Autodesk Inventor part; units mm, degrees
(part 8 of 13)
  line L2760 (6.8105, 15.183) -> (1.0789, 15.183)
  arc A2760 (1.0789, 15.183) -> (1.0789, 15.057) centre (1.0789, 15.12) ccw
  line L2761 (8.5894, 15.057) -> (17.121, 15.057)
  arc A2761 (17.121, 15.057) -> (17.121, 15.183) centre (17.121, 15.12) ccw
  line L2762 (17.121, 15.183) -> (8.5894, 15.183)
  arc A2762 (8.5894, 15.183) -> (8.5894, 15.057) centre (8.5894, 15.12) ccw
  line L2763 (1.0789, 15.183) -> (6.9365, 15.183)
  arc A2763 (6.9365, 15.183) -> (6.9365, 15.309) centre (6.9365, 15.246) ccw
  line L2764 (6.9365, 15.309) -> (1.0789, 15.309)
  arc A2764 (1.0789, 15.309) -> (1.0789, 15.183) centre (1.0789, 15.246) ccw
  line L2765 (8.4634, 15.183) -> (17.121, 15.183)
  arc A2765 (17.121, 15.183) -> (17.121, 15.309) centre (17.121, 15.246) ccw
  line L2766 (17.121, 15.309) -> (8.4634, 15.309)
  arc A2766 (8.4634, 15.309) -> (8.4634, 15.183) centre (8.4634, 15.246) ccw
  line L2767 (1.0789, 15.309) -> (7.1747, 15.309)
  arc A2767 (7.1747, 15.309) -> (7.1747, 15.435) centre (7.1747, 15.372) ccw
  line L2768 (7.1747, 15.435) -> (1.0789, 15.435)
  arc A2768 (1.0789, 15.435) -> (1.0789, 15.309) centre (1.0789, 15.372) ccw
  line L2769 (8.2253, 15.309) -> (17.121, 15.309)
  arc A2769 (17.121, 15.309) -> (17.121, 15.435) centre (17.121, 15.372) ccw
  line L2770 (17.121, 15.435) -> (8.2253, 15.435)
  arc A2770 (8.2253, 15.435) -> (8.2253, 15.309) centre (8.2253, 15.372) ccw
  line L2771 (1.0789, 15.435) -> (17.121, 15.435)
  arc A2771 (17.121, 15.435) -> (17.121, 15.561) centre (17.121, 15.498) ccw
  line L2772 (17.121, 15.561) -> (1.0789, 15.561)
  arc A2772 (1.0789, 15.561) -> (1.0789, 15.435) centre (1.0789, 15.498) ccw
  line L2773 (1.0789, 15.561) -> (17.121, 15.561)
  arc A2773 (17.121, 15.561) -> (17.121, 15.687) centre (17.121, 15.624) ccw
  line L2774 (17.121, 15.687) -> (1.0789, 15.687)
  arc A2774 (1.0789, 15.687) -> (1.0789, 15.561) centre (1.0789, 15.624) ccw
  line L2775 (1.0789, 15.687) -> (17.121, 15.687)
  arc A2775 (17.121, 15.687) -> (17.121, 15.813) centre (17.121, 15.75) ccw
  line L2776 (17.121, 15.813) -> (1.0789, 15.813)
  arc A2776 (1.0789, 15.813) -> (1.0789, 15.687) centre (1.0789, 15.75) ccw
  line L2777 (1.0789, 15.813) -> (17.121, 15.813)
  arc A2777 (17.121, 15.813) -> (17.121, 15.939) centre (17.121, 15.876) ccw
  line L2778 (17.121, 15.939) -> (1.0789, 15.939)
  arc A2778 (1.0789, 15.939) -> (1.0789, 15.813) centre (1.0789, 15.876) ccw
  line L2779 (1.0789, 15.939) -> (17.121, 15.939)
  arc A2779 (17.121, 15.939) -> (17.121, 16.065) centre (17.121, 16.002) ccw
  line L2780 (17.121, 16.065) -> (1.0789, 16.065)
  arc A2780 (1.0789, 16.065) -> (1.0789, 15.939) centre (1.0789, 16.002) ccw
  line L2781 (1.0789, 16.065) -> (17.121, 16.065)
  arc A2781 (17.121, 16.065) -> (17.121, 16.191) centre (17.121, 16.128) ccw
  line L2782 (17.121, 16.191) -> (1.0789, 16.191)
  arc A2782 (1.0789, 16.191) -> (1.0789, 16.065) centre (1.0789, 16.128) ccw
  line L2783 (1.0789, 16.191) -> (17.121, 16.191)
  arc A2783 (17.121, 16.191) -> (17.121, 16.317) centre (17.121, 16.254) ccw
  line L2784 (17.121, 16.317) -> (1.0789, 16.317)
  arc A2784 (1.0789, 16.317) -> (1.0789, 16.191) centre (1.0789, 16.254) ccw
  line L2785 (1.0789, 16.317) -> (17.121, 16.317)
  arc A2785 (17.121, 16.317) -> (17.121, 16.443) centre (17.121, 16.38) ccw
  line L2786 (17.121, 16.443) -> (1.0789, 16.443)
  arc A2786 (1.0789, 16.443) -> (1.0789, 16.317) centre (1.0789, 16.38) ccw
  line L2787 (1.0789, 16.443) -> (17.121, 16.443)
  arc A2787 (17.121, 16.443) -> (17.121, 16.569) centre (17.121, 16.506) ccw
  line L2788 (17.121, 16.569) -> (1.0789, 16.569)
  arc A2788 (1.0789, 16.569) -> (1.0789, 16.443) centre (1.0789, 16.506) ccw
  line L2789 (1.0789, 16.569) -> (17.121, 16.569)
  arc A2789 (17.121, 16.569) -> (17.121, 16.695) centre (17.121, 16.632) ccw
  line L2790 (17.121, 16.695) -> (1.0789, 16.695)
  arc A2790 (1.0789, 16.695) -> (1.0789, 16.569) centre (1.0789, 16.632) ccw
  line L2791 (1.0789, 16.695) -> (17.121, 16.695)
  arc A2791 (17.121, 16.695) -> (17.121, 16.821) centre (17.121, 16.758) ccw
  line L2792 (17.121, 16.821) -> (1.0789, 16.821)
  arc A2792 (1.0789, 16.821) -> (1.0789, 16.695) centre (1.0789, 16.758) ccw
  line L2793 (1.0789, 16.821) -> (17.121, 16.821)
  arc A2793 (17.121, 16.821) -> (17.121, 16.947) centre (17.121, 16.884) ccw
  line L2794 (17.121, 16.947) -> (1.0789, 16.947)
  arc A2794 (1.0789, 16.947) -> (1.0789, 16.821) centre (1.0789, 16.884) ccw
  line L2795 (1.0789, 16.947) -> (17.121, 16.947)
  arc A2795 (17.121, 16.947) -> (17.121, 17.073) centre (17.121, 17.01) ccw
  line L2796 (17.121, 17.073) -> (1.0789, 17.073)
  arc A2796 (1.0789, 17.073) -> (1.0789, 16.947) centre (1.0789, 17.01) ccw
  line L2797 (1.0789, 17.073) -> (17.121, 17.073)
  arc A2797 (17.121, 17.073) -> (17.121, 17.199) centre (17.121, 17.136) ccw
  line L2798 (17.121, 17.199) -> (1.0789, 17.199)
  arc A2798 (1.0789, 17.199) -> (1.0789, 17.073) centre (1.0789, 17.136) ccw
  line L2799 (1.0789, 17.199) -> (17.121, 17.199)
  arc A2799 (17.121, 17.199) -> (17.121, 17.325) centre (17.121, 17.262) ccw
  line L2800 (17.121, 17.325) -> (1.0789, 17.325)
  arc A2800 (1.0789, 17.325) -> (1.0789, 17.199) centre (1.0789, 17.262) ccw
  line L2801 (1.0789, 17.325) -> (17.121, 17.325)
  arc A2801 (17.121, 17.325) -> (17.121, 17.451) centre (17.121, 17.388) ccw
  line L2802 (17.121, 17.451) -> (1.0789, 17.451)
  arc A2802 (1.0789, 17.451) -> (1.0789, 17.325) centre (1.0789, 17.388) ccw
  line L2803 (1.0789, 17.451) -> (17.121, 17.451)
  arc A2803 (17.121, 17.451) -> (17.121, 17.577) centre (17.121, 17.514) ccw
  line L2804 (17.121, 17.577) -> (1.0789, 17.577)
  arc A2804 (1.0789, 17.577) -> (1.0789, 17.451) centre (1.0789, 17.514) ccw
  line L2805 (1.0789, 17.577) -> (17.121, 17.577)
  arc A2805 (17.121, 17.577) -> (17.121, 17.703) centre (17.121, 17.64) ccw
  line L2806 (17.121, 17.703) -> (1.0789, 17.703)
  arc A2806 (1.0789, 17.703) -> (1.0789, 17.577) centre (1.0789, 17.64) ccw
  line L2807 (1.0789, 17.703) -> (17.121, 17.703)
  arc A2807 (17.121, 17.703) -> (17.121, 17.829) centre (17.121, 17.766) ccw
  line L2808 (17.121, 17.829) -> (1.0789, 17.829)
  arc A2808 (1.0789, 17.829) -> (1.0789, 17.703) centre (1.0789, 17.766) ccw
  line L2809 (1.0789, 17.829) -> (17.121, 17.829)
  arc A2809 (17.121, 17.829) -> (17.121, 17.955) centre (17.121, 17.892) ccw
  line L2810 (17.121, 17.955) -> (1.0789, 17.955)
  arc A2810 (1.0789, 17.955) -> (1.0789, 17.829) centre (1.0789, 17.892) ccw
  line L2811 (1.0789, 17.955) -> (7.2227, 17.955)
  arc A2811 (7.2227, 17.955) -> (7.2227, 18.081) centre (7.2227, 18.018) ccw
  line L2812 (7.2227, 18.081) -> (1.0789, 18.081)
  arc A2812 (1.0789, 18.081) -> (1.0789, 17.955) centre (1.0789, 18.018) ccw
  line L2813 (7.637, 17.955) -> (7.7628, 17.955)
  arc A2813 (7.7628, 17.955) -> (7.7628, 18.081) centre (7.7628, 18.018) ccw
  line L2814 (7.7628, 18.081) -> (7.637, 18.081)
  arc A2814 (7.637, 18.081) -> (7.637, 17.955) centre (7.637, 18.018) ccw
  line L2815 (8.1771, 17.955) -> (17.121, 17.955)
  arc A2815 (17.121, 17.955) -> (17.121, 18.081) centre (17.121, 18.018) ccw
  line L2816 (17.121, 18.081) -> (8.1771, 18.081)
  arc A2816 (8.1771, 18.081) -> (8.1771, 17.955) centre (8.1771, 18.018) ccw
  line L2817 (1.0789, 18.081) -> (6.9227, 18.081)
  arc A2817 (6.9227, 18.081) -> (6.9227, 18.207) centre (6.9227, 18.144) ccw
  line L2818 (6.9227, 18.207) -> (1.0789, 18.207)
  arc A2818 (1.0789, 18.207) -> (1.0789, 18.081) centre (1.0789, 18.144) ccw
  line L2819 (7.637, 18.081) -> (7.7628, 18.081)
  arc A2819 (7.7628, 18.081) -> (7.7628, 18.207) centre (7.7628, 18.144) ccw
  line L2820 (7.7628, 18.207) -> (7.637, 18.207)
  arc A2820 (7.637, 18.207) -> (7.637, 18.081) centre (7.637, 18.144) ccw
  line L2821 (8.4772, 18.081) -> (17.121, 18.081)
  arc A2821 (17.121, 18.081) -> (17.121, 18.207) centre (17.121, 18.144) ccw
  line L2822 (17.121, 18.207) -> (8.4772, 18.207)
  arc A2822 (8.4772, 18.207) -> (8.4772, 18.081) centre (8.4772, 18.144) ccw
  line L2823 (1.0789, 18.207) -> (6.7967, 18.207)
  arc A2823 (6.7967, 18.207) -> (6.7967, 18.333) centre (6.7967, 18.27) ccw
  line L2824 (6.7967, 18.333) -> (1.0789, 18.333)
  arc A2824 (1.0789, 18.333) -> (1.0789, 18.207) centre (1.0789, 18.27) ccw
  line L2825 (7.637, 18.207) -> (7.7628, 18.207)
  arc A2825 (7.7628, 18.207) -> (7.7628, 18.333) centre (7.7628, 18.27) ccw
  line L2826 (7.7628, 18.333) -> (7.637, 18.333)
  arc A2826 (7.637, 18.333) -> (7.637, 18.207) centre (7.637, 18.27) ccw
  line L2827 (8.6032, 18.207) -> (17.121, 18.207)
  arc A2827 (17.121, 18.207) -> (17.121, 18.333) centre (17.121, 18.27) ccw
  line L2828 (17.121, 18.333) -> (8.6032, 18.333)
  arc A2828 (8.6032, 18.333) -> (8.6032, 18.207) centre (8.6032, 18.27) ccw
  line L2829 (1.0789, 18.333) -> (1.3493, 18.333)
  arc A2829 (1.3493, 18.333) -> (1.3493, 18.459) centre (1.3493, 18.396) ccw
  line L2830 (1.3493, 18.459) -> (1.0789, 18.459)
  arc A2830 (1.0789, 18.459) -> (1.0789, 18.333) centre (1.0789, 18.396) ccw
  line L2831 (3.4506, 18.333) -> (6.6707, 18.333)
  arc A2831 (6.6707, 18.333) -> (6.6707, 18.459) centre (6.6707, 18.396) ccw
  line L2832 (6.6707, 18.459) -> (3.4506, 18.459)
  arc A2832 (3.4506, 18.459) -> (3.4506, 18.333) centre (3.4506, 18.396) ccw
  line L2833 (7.637, 18.333) -> (7.7628, 18.333)
  arc A2833 (7.7628, 18.333) -> (7.7628, 18.459) centre (7.7628, 18.396) ccw
  line L2834 (7.7628, 18.459) -> (7.637, 18.459)
  arc A2834 (7.637, 18.459) -> (7.637, 18.333) centre (7.637, 18.396) ccw
  line L2835 (8.7292, 18.333) -> (17.121, 18.333)
  arc A2835 (17.121, 18.333) -> (17.121, 18.459) centre (17.121, 18.396) ccw
  line L2836 (17.121, 18.459) -> (8.7292, 18.459)
  arc A2836 (8.7292, 18.459) -> (8.7292, 18.333) centre (8.7292, 18.396) ccw
  line L2837 (1.0789, 18.459) -> (1.2846, 18.459)
  arc A2837 (1.2846, 18.459) -> (1.2846, 18.585) centre (1.2846, 18.522) ccw
  line L2838 (1.2846, 18.585) -> (1.0789, 18.585)
  arc A2838 (1.0789, 18.585) -> (1.0789, 18.459) centre (1.0789, 18.522) ccw
  line L2839 (3.5153, 18.459) -> (6.5447, 18.459)
  arc A2839 (6.5447, 18.459) -> (6.5447, 18.585) centre (6.5447, 18.522) ccw
  line L2840 (6.5447, 18.585) -> (3.5153, 18.585)
  arc A2840 (3.5153, 18.585) -> (3.5153, 18.459) centre (3.5153, 18.522) ccw
  line L2841 (7.637, 18.459) -> (7.7628, 18.459)
  arc A2841 (7.7628, 18.459) -> (7.7628, 18.585) centre (7.7628, 18.522) ccw
  line L2842 (7.7628, 18.585) -> (7.637, 18.585)
  arc A2842 (7.637, 18.585) -> (7.637, 18.459) centre (7.637, 18.522) ccw
  line L2843 (8.8552, 18.459) -> (17.121, 18.459)
  arc A2843 (17.121, 18.459) -> (17.121, 18.585) centre (17.121, 18.522) ccw
  line L2844 (17.121, 18.585) -> (8.8552, 18.585)
  arc A2844 (8.8552, 18.585) -> (8.8552, 18.459) centre (8.8552, 18.522) ccw
  line L2845 (1.0789, 18.585) -> (1.2846, 18.585)
  arc A2845 (1.2846, 18.585) -> (1.2846, 18.711) centre (1.2846, 18.648) ccw
  line L2846 (1.2846, 18.711) -> (1.0789, 18.711)
  arc A2846 (1.0789, 18.711) -> (1.0789, 18.585) centre (1.0789, 18.648) ccw
  line L2847 (3.5153, 18.585) -> (6.4904, 18.585)
  arc A2847 (6.4904, 18.585) -> (6.4904, 18.711) centre (6.4904, 18.648) ccw
  line L2848 (6.4904, 18.711) -> (3.5153, 18.711)
  arc A2848 (3.5153, 18.711) -> (3.5153, 18.585) centre (3.5153, 18.648) ccw
  line L2849 (7.637, 18.585) -> (7.7628, 18.585)
  arc A2849 (7.7628, 18.585) -> (7.7628, 18.711) centre (7.7628, 18.648) ccw
  line L2850 (7.7628, 18.711) -> (7.637, 18.711)
  arc A2850 (7.637, 18.711) -> (7.637, 18.585) centre (7.637, 18.648) ccw
  line L2851 (8.9094, 18.585) -> (17.121, 18.585)
  arc A2851 (17.121, 18.585) -> (17.121, 18.711) centre (17.121, 18.648) ccw
  line L2852 (17.121, 18.711) -> (8.9094, 18.711)
  arc A2852 (8.9094, 18.711) -> (8.9094, 18.585) centre (8.9094, 18.648) ccw
  line L2853 (1.0789, 18.711) -> (1.2846, 18.711)
  arc A2853 (1.2846, 18.711) -> (1.2846, 18.837) centre (1.2846, 18.774) ccw
  line L2854 (1.2846, 18.837) -> (1.0789, 18.837)
  arc A2854 (1.0789, 18.837) -> (1.0789, 18.711) centre (1.0789, 18.774) ccw
  line L2855 (3.5153, 18.711) -> (6.4382, 18.711)
  arc A2855 (6.4382, 18.711) -> (6.4382, 18.837) centre (6.4382, 18.774) ccw
  line L2856 (6.4382, 18.837) -> (3.5153, 18.837)
  arc A2856 (3.5153, 18.837) -> (3.5153, 18.711) centre (3.5153, 18.774) ccw
  line L2857 (7.637, 18.711) -> (7.7628, 18.711)
  arc A2857 (7.7628, 18.711) -> (7.7628, 18.837) centre (7.7628, 18.774) ccw
  line L2858 (7.7628, 18.837) -> (7.637, 18.837)
  arc A2858 (7.637, 18.837) -> (7.637, 18.711) centre (7.637, 18.774) ccw
  line L2859 (8.9616, 18.711) -> (17.121, 18.711)
  arc A2859 (17.121, 18.711) -> (17.121, 18.837) centre (17.121, 18.774) ccw
  line L2860 (17.121, 18.837) -> (8.9616, 18.837)
  arc A2860 (8.9616, 18.837) -> (8.9616, 18.711) centre (8.9616, 18.774) ccw
  line L2861 (1.0789, 18.837) -> (1.2846, 18.837)
  arc A2861 (1.2846, 18.837) -> (1.2846, 18.963) centre (1.2846, 18.9) ccw
  line L2862 (1.2846, 18.963) -> (1.0789, 18.963)
  arc A2862 (1.0789, 18.963) -> (1.0789, 18.837) centre (1.0789, 18.9) ccw
  line L2863 (3.5153, 18.837) -> (6.386, 18.837)
  arc A2863 (6.386, 18.837) -> (6.386, 18.963) centre (6.386, 18.9) ccw
  line L2864 (6.386, 18.963) -> (3.5153, 18.963)
  arc A2864 (3.5153, 18.963) -> (3.5153, 18.837) centre (3.5153, 18.9) ccw
  line L2865 (7.637, 18.837) -> (7.7628, 18.837)
  arc A2865 (7.7628, 18.837) -> (7.7628, 18.963) centre (7.7628, 18.9) ccw
  line L2866 (7.7628, 18.963) -> (7.637, 18.963)
  arc A2866 (7.637, 18.963) -> (7.637, 18.837) centre (7.637, 18.9) ccw
  line L2867 (9.0138, 18.837) -> (17.121, 18.837)
  arc A2867 (17.121, 18.837) -> (17.121, 18.963) centre (17.121, 18.9) ccw
  line L2868 (17.121, 18.963) -> (9.0138, 18.963)
  arc A2868 (9.0138, 18.963) -> (9.0138, 18.837) centre (9.0138, 18.9) ccw
  line L2869 (1.0789, 18.963) -> (1.2846, 18.963)
  arc A2869 (1.2846, 18.963) -> (1.2846, 19.089) centre (1.2846, 19.026) ccw
  line L2870 (1.2846, 19.089) -> (1.0789, 19.089)
  arc A2870 (1.0789, 19.089) -> (1.0789, 18.963) centre (1.0789, 19.026) ccw
  line L2871 (3.5153, 18.963) -> (6.3338, 18.963)
  arc A2871 (6.3338, 18.963) -> (6.3338, 19.089) centre (6.3338, 19.026) ccw
  line L2872 (6.3338, 19.089) -> (3.5153, 19.089)
  arc A2872 (3.5153, 19.089) -> (3.5153, 18.963) centre (3.5153, 19.026) ccw
  line L2873 (7.637, 18.963) -> (7.7628, 18.963)
  arc A2873 (7.7628, 18.963) -> (7.7632, 19.089) centre (7.763, 19.026) ccw
  line L2874 (7.7632, 19.089) -> (7.6374, 19.089)
  arc A2874 (7.6374, 19.089) -> (7.637, 18.963) centre (7.6372, 19.026) ccw
  line L2875 (9.066, 18.963) -> (17.121, 18.963)
  arc A2875 (17.121, 18.963) -> (17.1212, 19.0315) centre (17.174, 18.9971) ccw
  line L2876 (17.1212, 19.0315) -> (9.0664, 19.089)
  arc A2876 (9.0664, 19.089) -> (9.066, 18.963) centre (9.0662, 19.026) ccw
  line L2877 (1.0789, 19.089) -> (1.2846, 19.089)
  arc A2877 (1.2846, 19.089) -> (1.2846, 19.215) centre (1.2846, 19.152) ccw
  line L2878 (1.2846, 19.215) -> (1.0789, 19.215)
  arc A2878 (1.0789, 19.215) -> (1.0789, 19.089) centre (1.0789, 19.152) ccw
  line L2879 (3.5153, 19.089) -> (6.333, 19.089)
  arc A2879 (6.333, 19.089) -> (6.3334, 19.215) centre (6.3334, 19.152) ccw
  line L2880 (6.3334, 19.215) -> (3.5157, 19.215)
  arc A2880 (3.5157, 19.215) -> (3.5153, 19.089) centre (3.5155, 19.152) ccw
  line L2881 (7.6374, 19.089) -> (7.7632, 19.089)
  arc A2881 (7.7632, 19.089) -> (7.7632, 19.215) centre (7.7632, 19.152) ccw
  line L2882 (7.7632, 19.215) -> (7.6374, 19.215)
  arc A2882 (7.6374, 19.215) -> (7.6374, 19.089) centre (7.6374, 19.152) ccw
  line L2883 (9.0673, 19.089) -> (17.1212, 19.0315)
  arc A2883 (17.1212, 19.0315) -> (17.1214, 19.215) centre (17.1213, 19.1232) ccw
  line L2884 (17.1214, 19.215) -> (9.0673, 19.215)
  arc A2884 (9.0673, 19.215) -> (9.0673, 19.089) centre (9.0673, 19.152) ccw
  line L2885 (1.0789, 19.215) -> (1.2846, 19.215)
  arc A2885 (1.2846, 19.215) -> (1.2846, 19.341) centre (1.2846, 19.278) ccw
  line L2886 (1.2846, 19.341) -> (1.0789, 19.341)
  arc A2886 (1.0789, 19.341) -> (1.0789, 19.215) centre (1.0789, 19.278) ccw
  line L2887 (3.5157, 19.215) -> (7.6369, 19.215)
  arc A2887 (7.6369, 19.215) -> (7.6369, 19.341) centre (7.6369, 19.278) ccw
  line L2888 (7.6369, 19.341) -> (3.5157, 19.341)
  arc A2888 (3.5157, 19.341) -> (3.5157, 19.215) centre (3.5157, 19.278) ccw
  line L2889 (7.7638, 19.215) -> (17.1214, 19.215)
  arc A2889 (17.1214, 19.215) -> (17.1214, 19.341) centre (17.1214, 19.278) ccw
  line L2890 (17.1214, 19.341) -> (7.7638, 19.341)
  arc A2890 (7.7638, 19.341) -> (7.7638, 19.215) centre (7.7638, 19.278) ccw
  line L2891 (1.0789, 19.341) -> (1.2846, 19.341)
  arc A2891 (1.2846, 19.341) -> (1.2846, 19.467) centre (1.2846, 19.404) ccw
  line L2892 (1.2846, 19.467) -> (1.0789, 19.467)
  arc A2892 (1.0789, 19.467) -> (1.0789, 19.341) centre (1.0789, 19.404) ccw
  line L2893 (3.5157, 19.341) -> (6.3334, 19.341)
  arc A2893 (6.3334, 19.341) -> (6.3334, 19.467) centre (6.3334, 19.404) ccw
  line L2894 (6.3334, 19.467) -> (3.5157, 19.467)
  arc A2894 (3.5157, 19.467) -> (3.5157, 19.341) centre (3.5157, 19.404) ccw
  line L2895 (7.6374, 19.341) -> (7.7632, 19.341)
  arc A2895 (7.7632, 19.341) -> (7.7632, 19.467) centre (7.7632, 19.404) ccw
  line L2896 (7.7632, 19.467) -> (7.6374, 19.467)
  arc A2896 (7.6374, 19.467) -> (7.6374, 19.341) centre (7.6374, 19.404) ccw
  line L2897 (9.0673, 19.341) -> (17.1214, 19.341)
  arc A2897 (17.1214, 19.341) -> (17.1214, 19.467) centre (17.1214, 19.404) ccw
  line L2898 (17.1214, 19.467) -> (9.0673, 19.467)
  arc A2898 (9.0673, 19.467) -> (9.0673, 19.341) centre (9.0673, 19.404) ccw
  line L2899 (1.0789, 19.467) -> (1.2846, 19.467)
  arc A2899 (1.2846, 19.467) -> (1.2846, 19.593) centre (1.2846, 19.53) ccw
  line L2900 (1.2846, 19.593) -> (1.0789, 19.593)
  arc A2900 (1.0789, 19.593) -> (1.0789, 19.467) centre (1.0789, 19.53) ccw
  line L2901 (3.5157, 19.467) -> (6.3334, 19.467)
  arc A2901 (6.3334, 19.467) -> (6.3334, 19.593) centre (6.3334, 19.53) ccw
  line L2902 (6.3334, 19.593) -> (3.5157, 19.593)
  arc A2902 (3.5157, 19.593) -> (3.5157, 19.467) centre (3.5157, 19.53) ccw
  line L2903 (7.6374, 19.467) -> (7.7632, 19.467)
  arc A2903 (7.7632, 19.467) -> (7.7632, 19.593) centre (7.7632, 19.53) ccw
  line L2904 (7.7632, 19.593) -> (7.6374, 19.593)
  arc A2904 (7.6374, 19.593) -> (7.6374, 19.467) centre (7.6374, 19.53) ccw
  line L2905 (9.0673, 19.467) -> (17.1214, 19.467)
  arc A2905 (17.1214, 19.467) -> (17.121, 19.593) centre (17.1212, 19.53) ccw
  line L2906 (17.121, 19.593) -> (9.0669, 19.593)
  arc A2906 (9.0669, 19.593) -> (9.0673, 19.467) centre (9.0671, 19.53) ccw
  line L2907 (1.0789, 19.593) -> (1.2846, 19.593)
  arc A2907 (1.2846, 19.593) -> (1.2846, 19.719) centre (1.2846, 19.656) ccw
  line L2908 (1.2846, 19.719) -> (1.0789, 19.719)
  arc A2908 (1.0789, 19.719) -> (1.0789, 19.593) centre (1.0789, 19.656) ccw
  line L2909 (3.5157, 19.593) -> (6.3683, 19.593)
  arc A2909 (6.3683, 19.593) -> (6.3683, 19.719) centre (6.3683, 19.656) ccw
  line L2910 (6.3683, 19.719) -> (3.5157, 19.719)
  arc A2910 (3.5157, 19.719) -> (3.5157, 19.593) centre (3.5157, 19.656) ccw
  line L2911 (7.6374, 19.593) -> (7.7632, 19.593)
  arc A2911 (7.7632, 19.593) -> (7.7632, 19.719) centre (7.7632, 19.656) ccw
  line L2912 (7.7632, 19.719) -> (7.6374, 19.719)
  arc A2912 (7.6374, 19.719) -> (7.6374, 19.593) centre (7.6374, 19.656) ccw
  line L2913 (9.0321, 19.593) -> (17.121, 19.593)
  arc A2913 (17.121, 19.593) -> (17.121, 19.719) centre (17.121, 19.656) ccw
  line L2914 (17.121, 19.719) -> (9.0321, 19.719)
  arc A2914 (9.0321, 19.719) -> (9.0321, 19.593) centre (9.0321, 19.656) ccw
  line L2915 (1.0789, 19.719) -> (1.2846, 19.719)
  arc A2915 (1.2846, 19.719) -> (1.2846, 19.845) centre (1.2846, 19.782) ccw
  line L2916 (1.2846, 19.845) -> (1.0789, 19.845)
  arc A2916 (1.0789, 19.845) -> (1.0789, 19.719) centre (1.0789, 19.782) ccw
  line L2917 (3.5157, 19.719) -> (6.4205, 19.719)
  arc A2917 (6.4205, 19.719) -> (6.4205, 19.845) centre (6.4205, 19.782) ccw
  line L2918 (6.4205, 19.845) -> (3.5157, 19.845)
  arc A2918 (3.5157, 19.845) -> (3.5157, 19.719) centre (3.5157, 19.782) ccw
  line L2919 (7.6374, 19.719) -> (7.7632, 19.719)
  arc A2919 (7.7632, 19.719) -> (7.7632, 19.845) centre (7.7632, 19.782) ccw
  line L2920 (7.7632, 19.845) -> (7.6374, 19.845)
  arc A2920 (7.6374, 19.845) -> (7.6374, 19.719) centre (7.6374, 19.782) ccw
  line L2921 (8.9799, 19.719) -> (17.121, 19.719)
  arc A2921 (17.121, 19.719) -> (17.121, 19.845) centre (17.121, 19.782) ccw
  line L2922 (17.121, 19.845) -> (8.9799, 19.845)
  arc A2922 (8.9799, 19.845) -> (8.9799, 19.719) centre (8.9799, 19.782) ccw
  line L2923 (1.0789, 19.845) -> (1.2846, 19.845)
  arc A2923 (1.2846, 19.845) -> (1.2846, 19.971) centre (1.2846, 19.908) ccw
  line L2924 (1.2846, 19.971) -> (1.0789, 19.971)
  arc A2924 (1.0789, 19.971) -> (1.0789, 19.845) centre (1.0789, 19.908) ccw
  line L2925 (3.5157, 19.845) -> (6.4727, 19.845)
  arc A2925 (6.4727, 19.845) -> (6.4727, 19.971) centre (6.4727, 19.908) ccw
  line L2926 (6.4727, 19.971) -> (3.5157, 19.971)
  arc A2926 (3.5157, 19.971) -> (3.5157, 19.845) centre (3.5157, 19.908) ccw
  line L2927 (7.6374, 19.845) -> (7.7632, 19.845)
  arc A2927 (7.7632, 19.845) -> (7.7632, 19.971) centre (7.7632, 19.908) ccw
  line L2928 (7.7632, 19.971) -> (7.6374, 19.971)
  arc A2928 (7.6374, 19.971) -> (7.6374, 19.845) centre (7.6374, 19.908) ccw
  line L2929 (8.9277, 19.845) -> (17.121, 19.845)
  arc A2929 (17.121, 19.845) -> (17.121, 19.971) centre (17.121, 19.908) ccw
  line L2930 (17.121, 19.971) -> (8.9277, 19.971)
  arc A2930 (8.9277, 19.971) -> (8.9277, 19.845) centre (8.9277, 19.908) ccw
  line L2931 (1.0789, 19.971) -> (1.2846, 19.971)
  arc A2931 (1.2846, 19.971) -> (1.2846, 20.097) centre (1.2846, 20.034) ccw
  line L2932 (1.2846, 20.097) -> (1.0789, 20.097)
  arc A2932 (1.0789, 20.097) -> (1.0789, 19.971) centre (1.0789, 20.034) ccw
  line L2933 (3.5157, 19.971) -> (6.5249, 19.971)
  arc A2933 (6.5249, 19.971) -> (6.5249, 20.097) centre (6.5249, 20.034) ccw
  line L2934 (6.5249, 20.097) -> (3.5157, 20.097)
  arc A2934 (3.5157, 20.097) -> (3.5157, 19.971) centre (3.5157, 20.034) ccw
  line L2935 (7.6374, 19.971) -> (7.7632, 19.971)
  arc A2935 (7.7632, 19.971) -> (7.7632, 20.097) centre (7.7632, 20.034) ccw
  line L2936 (7.7632, 20.097) -> (7.6374, 20.097)
  arc A2936 (7.6374, 20.097) -> (7.6374, 19.971) centre (7.6374, 20.034) ccw
  line L2937 (8.8755, 19.971) -> (17.121, 19.971)
  arc A2937 (17.121, 19.971) -> (17.121, 20.097) centre (17.121, 20.034) ccw
  line L2938 (17.121, 20.097) -> (8.8755, 20.097)
  arc A2938 (8.8755, 20.097) -> (8.8755, 19.971) centre (8.8755, 20.034) ccw
  line L2939 (1.0789, 20.097) -> (1.2846, 20.097)
  arc A2939 (1.2846, 20.097) -> (1.2846, 20.223) centre (1.2846, 20.16) ccw
  line L2940 (1.2846, 20.223) -> (1.0789, 20.223)
  arc A2940 (1.0789, 20.223) -> (1.0789, 20.097) centre (1.0789, 20.16) ccw
  line L2941 (3.5157, 20.097) -> (6.6272, 20.097)
  arc A2941 (6.6272, 20.097) -> (6.6272, 20.223) centre (6.6272, 20.16) ccw
  line L2942 (6.6272, 20.223) -> (3.5157, 20.223)
  arc A2942 (3.5157, 20.223) -> (3.5157, 20.097) centre (3.5157, 20.16) ccw
  line L2943 (7.6374, 20.097) -> (7.7632, 20.097)
  arc A2943 (7.7632, 20.097) -> (7.7632, 20.223) centre (7.7632, 20.16) ccw
  line L2944 (7.7632, 20.223) -> (7.6374, 20.223)
  arc A2944 (7.6374, 20.223) -> (7.6374, 20.097) centre (7.6374, 20.16) ccw
  line L2945 (8.7731, 20.097) -> (17.121, 20.097)
  arc A2945 (17.121, 20.097) -> (17.121, 20.223) centre (17.121, 20.16) ccw
  line L2946 (17.121, 20.223) -> (8.7731, 20.223)
  arc A2946 (8.7731, 20.223) -> (8.7731, 20.097) centre (8.7731, 20.16) ccw
  line L2947 (1.0789, 20.223) -> (1.2846, 20.223)
  arc A2947 (1.2846, 20.223) -> (1.2846, 20.349) centre (1.2846, 20.286) ccw
  line L2948 (1.2846, 20.349) -> (1.0789, 20.349)
  arc A2948 (1.0789, 20.349) -> (1.0789, 20.223) centre (1.0789, 20.286) ccw
  line L2949 (3.5157, 20.223) -> (6.7532, 20.223)
  arc A2949 (6.7532, 20.223) -> (6.7532, 20.349) centre (6.7532, 20.286) ccw
  line L2950 (6.7532, 20.349) -> (3.5157, 20.349)
  arc A2950 (3.5157, 20.349) -> (3.5157, 20.223) centre (3.5157, 20.286) ccw
  line L2951 (7.6374, 20.223) -> (7.7632, 20.223)
  arc A2951 (7.7632, 20.223) -> (7.7632, 20.349) centre (7.7632, 20.286) ccw
  line L2952 (7.7632, 20.349) -> (7.6374, 20.349)
  arc A2952 (7.6374, 20.349) -> (7.6374, 20.223) centre (7.6374, 20.286) ccw
  line L2953 (8.6471, 20.223) -> (17.121, 20.223)
  arc A2953 (17.121, 20.223) -> (17.121, 20.349) centre (17.121, 20.286) ccw
  line L2954 (17.121, 20.349) -> (8.6471, 20.349)
  arc A2954 (8.6471, 20.349) -> (8.6471, 20.223) centre (8.6471, 20.286) ccw
  line L2955 (1.0789, 20.349) -> (1.2846, 20.349)
  arc A2955 (1.2846, 20.349) -> (1.2846, 20.475) centre (1.2846, 20.412) ccw
  line L2956 (1.2846, 20.475) -> (1.0789, 20.475)
  arc A2956 (1.0789, 20.475) -> (1.0789, 20.349) centre (1.0789, 20.412) ccw
  line L2957 (3.5157, 20.349) -> (6.8792, 20.349)
  arc A2957 (6.8792, 20.349) -> (6.8788, 20.475) centre (6.879, 20.412) ccw
  line L2958 (6.8788, 20.475) -> (3.5153, 20.475)
  arc A2958 (3.5153, 20.475) -> (3.5157, 20.349) centre (3.5155, 20.412) ccw
  line L2959 (7.6374, 20.349) -> (7.7632, 20.349)
  arc A2959 (7.7632, 20.349) -> (7.7632, 20.475) centre (7.7632, 20.412) ccw
  line L2960 (7.7632, 20.475) -> (7.6374, 20.475)
  arc A2960 (7.6374, 20.475) -> (7.6374, 20.349) centre (7.6374, 20.412) ccw
  line L2961 (8.5211, 20.349) -> (17.121, 20.349)
  arc A2961 (17.121, 20.349) -> (17.121, 20.475) centre (17.121, 20.412) ccw
  line L2962 (17.121, 20.475) -> (8.5211, 20.475)
  arc A2962 (8.5211, 20.475) -> (8.5211, 20.349) centre (8.5211, 20.412) ccw
  line L2963 (1.0789, 20.475) -> (1.3834, 20.475)
  arc A2963 (1.3834, 20.475) -> (1.3834, 20.601) centre (1.3834, 20.538) ccw
  line L2964 (1.3834, 20.601) -> (1.0789, 20.601)
  arc A2964 (1.0789, 20.601) -> (1.0789, 20.475) centre (1.0789, 20.538) ccw
  line L2965 (3.4165, 20.475) -> (7.1169, 20.475)
  arc A2965 (7.1169, 20.475) -> (7.1169, 20.601) centre (7.1169, 20.538) ccw
  line L2966 (7.1169, 20.601) -> (3.4165, 20.601)
  arc A2966 (3.4165, 20.601) -> (3.4165, 20.475) centre (3.4165, 20.538) ccw
  line L2967 (7.6374, 20.475) -> (7.7632, 20.475)
  arc A2967 (7.7632, 20.475) -> (7.7632, 20.601) centre (7.7632, 20.538) ccw
  line L2968 (7.7632, 20.601) -> (7.6374, 20.601)
  arc A2968 (7.6374, 20.601) -> (7.6374, 20.475) centre (7.6374, 20.538) ccw
  line L2969 (8.2831, 20.475) -> (17.121, 20.475)
  arc A2969 (17.121, 20.475) -> (17.121, 20.601) centre (17.121, 20.538) ccw
  line L2970 (17.121, 20.601) -> (8.2831, 20.601)
  arc A2970 (8.2831, 20.601) -> (8.2831, 20.475) centre (8.2831, 20.538) ccw
  line L2971 (1.0789, 20.601) -> (7.421, 20.601)
  arc A2971 (7.421, 20.601) -> (7.421, 20.727) centre (7.421, 20.664) ccw
  line L2972 (7.421, 20.727) -> (1.0789, 20.727)
  arc A2972 (1.0789, 20.727) -> (1.0789, 20.601) centre (1.0789, 20.664) ccw
  line L2973 (7.6374, 20.601) -> (7.7632, 20.601)
  arc A2973 (7.7632, 20.601) -> (7.7628, 20.727) centre (7.763, 20.664) ccw
  line L2974 (7.7628, 20.727) -> (7.637, 20.727)
  arc A2974 (7.637, 20.727) -> (7.6374, 20.601) centre (7.6372, 20.664) ccw
  line L2975 (7.979, 20.601) -> (17.121, 20.601)
  arc A2975 (17.121, 20.601) -> (17.121, 20.727) centre (17.121, 20.664) ccw
  line L2976 (17.121, 20.727) -> (7.979, 20.727)
  arc A2976 (7.979, 20.727) -> (7.979, 20.601) centre (7.979, 20.664) ccw
  line L2977 (1.0789, 20.727) -> (17.121, 20.727)
  arc A2977 (17.121, 20.727) -> (17.121, 20.853) centre (17.121, 20.79) ccw
  line L2978 (17.121, 20.853) -> (1.0789, 20.853)
  arc A2978 (1.0789, 20.853) -> (1.0789, 20.727) centre (1.0789, 20.79) ccw
  line L2979 (1.0789, 20.853) -> (17.121, 20.853)
  arc A2979 (17.121, 20.853) -> (17.121, 20.979) centre (17.121, 20.916) ccw
  line L2980 (17.121, 20.979) -> (1.0789, 20.979)
  arc A2980 (1.0789, 20.979) -> (1.0789, 20.853) centre (1.0789, 20.916) ccw
  line L2981 (1.0789, 20.979) -> (17.121, 20.979)
  arc A2981 (17.121, 20.979) -> (17.121, 21.105) centre (17.121, 21.042) ccw
  line L2982 (17.121, 21.105) -> (1.0789, 21.105)
  arc A2982 (1.0789, 21.105) -> (1.0789, 20.979) centre (1.0789, 21.042) ccw
  line L2983 (1.0789, 21.105) -> (17.121, 21.105)
  arc A2983 (17.121, 21.105) -> (17.121, 21.231) centre (17.121, 21.168) ccw
  line L2984 (17.121, 21.231) -> (1.0789, 21.231)
  arc A2984 (1.0789, 21.231) -> (1.0789, 21.105) centre (1.0789, 21.168) ccw
  line L2985 (1.0789, 21.231) -> (17.121, 21.231)
  arc A2985 (17.121, 21.231) -> (17.121, 21.357) centre (17.121, 21.294) ccw
  line L2986 (17.121, 21.357) -> (1.0789, 21.357)
  arc A2986 (1.0789, 21.357) -> (1.0789, 21.231) centre (1.0789, 21.294) ccw
  line L2987 (1.0789, 21.357) -> (17.121, 21.357)
  arc A2987 (17.121, 21.357) -> (17.121, 21.483) centre (17.121, 21.42) ccw
  line L2988 (17.121, 21.483) -> (1.0789, 21.483)
  arc A2988 (1.0789, 21.483) -> (1.0789, 21.357) centre (1.0789, 21.42) ccw
  line L2989 (1.0789, 21.483) -> (17.121, 21.483)
  arc A2989 (17.121, 21.483) -> (17.121, 21.609) centre (17.121, 21.546) ccw
  line L2990 (17.121, 21.609) -> (1.0789, 21.609)
  arc A2990 (1.0789, 21.609) -> (1.0789, 21.483) centre (1.0789, 21.546) ccw
  line L2991 (1.0789, 21.609) -> (17.121, 21.609)
  arc A2991 (17.121, 21.609) -> (17.121, 21.735) centre (17.121, 21.672) ccw
  line L2992 (17.121, 21.735) -> (1.0789, 21.735)
  arc A2992 (1.0789, 21.735) -> (1.0789, 21.609) centre (1.0789, 21.672) ccw
  line L2993 (1.0789, 21.735) -> (2.0009, 21.735)
  arc A2993 (2.0009, 21.735) -> (2.0009, 21.861) centre (2.0009, 21.798) ccw
  line L2994 (2.0009, 21.861) -> (1.0789, 21.861)
  arc A2994 (1.0789, 21.861) -> (1.0789, 21.735) centre (1.0789, 21.798) ccw
  line L2995 (2.337, 21.735) -> (2.4628, 21.735)
  arc A2995 (2.4628, 21.735) -> (2.4628, 21.861) centre (2.4628, 21.798) ccw
  line L2996 (2.4628, 21.861) -> (2.337, 21.861)
  arc A2996 (2.337, 21.861) -> (2.337, 21.735) centre (2.337, 21.798) ccw
  line L2997 (2.7989, 21.735) -> (17.121, 21.735)
  arc A2997 (17.121, 21.735) -> (17.121, 21.861) centre (17.121, 21.798) ccw
  line L2998 (17.121, 21.861) -> (2.7989, 21.861)
  arc A2998 (2.7989, 21.861) -> (2.7989, 21.735) centre (2.7989, 21.798) ccw
  line L2999 (1.0789, 21.861) -> (1.7049, 21.861)
  arc A2999 (1.7049, 21.861) -> (1.7049, 21.987) centre (1.7049, 21.924) ccw
  line L3000 (1.7049, 21.987) -> (1.0789, 21.987)
  arc A3000 (1.0789, 21.987) -> (1.0789, 21.861) centre (1.0789, 21.924) ccw
  line L3001 (2.337, 21.861) -> (2.4628, 21.861)
  arc A3001 (2.4628, 21.861) -> (2.4628, 21.987) centre (2.4628, 21.924) ccw
  line L3002 (2.4628, 21.987) -> (2.337, 21.987)
  arc A3002 (2.337, 21.987) -> (2.337, 21.861) centre (2.337, 21.924) ccw
  line L3003 (3.095, 21.861) -> (17.121, 21.861)
  arc A3003 (17.121, 21.861) -> (17.121, 21.987) centre (17.121, 21.924) ccw
  line L3004 (17.121, 21.987) -> (3.095, 21.987)
  arc A3004 (3.095, 21.987) -> (3.095, 21.861) centre (3.095, 21.924) ccw
  line L3005 (1.0789, 21.987) -> (1.5789, 21.987)
  arc A3005 (1.5789, 21.987) -> (1.5789, 22.113) centre (1.5789, 22.05) ccw
  line L3006 (1.5789, 22.113) -> (1.0789, 22.113)
  arc A3006 (1.0789, 22.113) -> (1.0789, 21.987) centre (1.0789, 22.05) ccw
  line L3007 (2.337, 21.987) -> (2.4628, 21.987)
  arc A3007 (2.4628, 21.987) -> (2.4628, 22.113) centre (2.4628, 22.05) ccw
  line L3008 (2.4628, 22.113) -> (2.337, 22.113)
  arc A3008 (2.337, 22.113) -> (2.337, 21.987) centre (2.337, 22.05) ccw
  line L3009 (3.221, 21.987) -> (17.121, 21.987)
  arc A3009 (17.121, 21.987) -> (17.121, 22.113) centre (17.121, 22.05) ccw
  line L3010 (17.121, 22.113) -> (3.221, 22.113)
  arc A3010 (3.221, 22.113) -> (3.221, 21.987) centre (3.221, 22.05) ccw
  line L3011 (1.0789, 22.113) -> (1.4529, 22.113)
  arc A3011 (1.4529, 22.113) -> (1.4529, 22.239) centre (1.4529, 22.176) ccw
  line L3012 (1.4529, 22.239) -> (1.0789, 22.239)
  arc A3012 (1.0789, 22.239) -> (1.0789, 22.113) centre (1.0789, 22.176) ccw
  line L3013 (2.337, 22.113) -> (2.4628, 22.113)
  arc A3013 (2.4628, 22.113) -> (2.4628, 22.239) centre (2.4628, 22.176) ccw
  line L3014 (2.4628, 22.239) -> (2.337, 22.239)
  arc A3014 (2.337, 22.239) -> (2.337, 22.113) centre (2.337, 22.176) ccw
  line L3015 (3.347, 22.113) -> (17.121, 22.113)
  arc A3015 (17.121, 22.113) -> (17.121, 22.239) centre (17.121, 22.176) ccw
  line L3016 (17.121, 22.239) -> (3.347, 22.239)
  arc A3016 (3.347, 22.239) -> (3.347, 22.113) centre (3.347, 22.176) ccw
  line L3017 (1.0789, 22.239) -> (1.3511, 22.239)
  arc A3017 (1.3511, 22.239) -> (1.3511, 22.365) centre (1.3511, 22.302) ccw
  line L3018 (1.3511, 22.365) -> (1.0789, 22.365)
  arc A3018 (1.0789, 22.365) -> (1.0789, 22.239) centre (1.0789, 22.302) ccw
  line L3019 (2.337, 22.239) -> (2.4628, 22.239)
  arc A3019 (2.4628, 22.239) -> (2.4628, 22.365) centre (2.4628, 22.302) ccw
  line L3020 (2.4628, 22.365) -> (2.337, 22.365)
  arc A3020 (2.337, 22.365) -> (2.337, 22.239) centre (2.337, 22.302) ccw
  line L3021 (3.4487, 22.239) -> (17.121, 22.239)
  arc A3021 (17.121, 22.239) -> (17.121, 22.365) centre (17.121, 22.302) ccw
  line L3022 (17.121, 22.365) -> (3.4487, 22.365)
  arc A3022 (3.4487, 22.365) -> (3.4487, 22.239) centre (3.4487, 22.302) ccw
  line L3023 (1.0789, 22.365) -> (1.2989, 22.365)
  arc A3023 (1.2989, 22.365) -> (1.2989, 22.491) centre (1.2989, 22.428) ccw
  line L3024 (1.2989, 22.491) -> (1.0789, 22.491)
  arc A3024 (1.0789, 22.491) -> (1.0789, 22.365) centre (1.0789, 22.428) ccw
  line L3025 (2.337, 22.365) -> (2.4628, 22.365)
  arc A3025 (2.4628, 22.365) -> (2.4628, 22.491) centre (2.4628, 22.428) ccw
  line L3026 (2.4628, 22.491) -> (2.337, 22.491)
  arc A3026 (2.337, 22.491) -> (2.337, 22.365) centre (2.337, 22.428) ccw
  line L3027 (3.5009, 22.365) -> (17.121, 22.365)
  arc A3027 (17.121, 22.365) -> (17.121, 22.491) centre (17.121, 22.428) ccw
  line L3028 (17.121, 22.491) -> (3.5009, 22.491)
  arc A3028 (3.5009, 22.491) -> (3.5009, 22.365) centre (3.5009, 22.428) ccw
  line L3029 (1.0789, 22.491) -> (1.2467, 22.491)
  arc A3029 (1.2467, 22.491) -> (1.2467, 22.617) centre (1.2467, 22.554) ccw
  line L3030 (1.2467, 22.617) -> (1.0789, 22.617)
  arc A3030 (1.0789, 22.617) -> (1.0789, 22.491) centre (1.0789, 22.554) ccw
  line L3031 (2.337, 22.491) -> (2.4628, 22.491)
  arc A3031 (2.4628, 22.491) -> (2.4628, 22.617) centre (2.4628, 22.554) ccw
  line L3032 (2.4628, 22.617) -> (2.337, 22.617)
  arc A3032 (2.337, 22.617) -> (2.337, 22.491) centre (2.337, 22.554) ccw
  line L3033 (3.5531, 22.491) -> (17.121, 22.491)
  arc A3033 (17.121, 22.491) -> (17.121, 22.617) centre (17.121, 22.554) ccw
  line L3034 (17.121, 22.617) -> (3.5531, 22.617)
  arc A3034 (3.5531, 22.617) -> (3.5531, 22.491) centre (3.5531, 22.554) ccw
  line L3035 (1.0789, 22.617) -> (1.1945, 22.617)
  arc A3035 (1.1945, 22.617) -> (1.1945, 22.743) centre (1.1945, 22.68) ccw
  line L3036 (1.1945, 22.743) -> (1.0789, 22.743)
  arc A3036 (1.0789, 22.743) -> (1.0789, 22.617) centre (1.0789, 22.68) ccw
  line L3037 (2.337, 22.617) -> (2.4628, 22.617)
  arc A3037 (2.4628, 22.617) -> (2.4628, 22.743) centre (2.4628, 22.68) ccw
  line L3038 (2.4628, 22.743) -> (2.337, 22.743)
  arc A3038 (2.337, 22.743) -> (2.337, 22.617) centre (2.337, 22.68) ccw
  line L3039 (3.6053, 22.617) -> (17.121, 22.617)
  arc A3039 (17.121, 22.617) -> (17.121, 22.743) centre (17.121, 22.68) ccw
  line L3040 (17.121, 22.743) -> (3.6053, 22.743)
  arc A3040 (3.6053, 22.743) -> (3.6053, 22.617) centre (3.6053, 22.68) ccw
  line L3041 (1.0789, 22.743) -> (1.183, 22.743)
  arc A3041 (1.183, 22.743) -> (1.183, 22.869) centre (1.183, 22.806) ccw
  line L3042 (1.183, 22.869) -> (1.0789, 22.869)
  arc A3042 (1.0789, 22.869) -> (1.0789, 22.743) centre (1.0789, 22.806) ccw
  line L3043 (2.337, 22.743) -> (2.4628, 22.743)
  arc A3043 (2.4628, 22.743) -> (2.4628, 22.869) centre (2.4628, 22.806) ccw
  line L3044 (2.4628, 22.869) -> (2.337, 22.869)
  arc A3044 (2.337, 22.869) -> (2.337, 22.743) centre (2.337, 22.806) ccw
  line L3045 (3.6169, 22.743) -> (17.121, 22.743)
  arc A3045 (17.121, 22.743) -> (17.121, 22.869) centre (17.121, 22.806) ccw
  line L3046 (17.121, 22.869) -> (3.6169, 22.869)
  arc A3046 (3.6169, 22.869) -> (3.6169, 22.743) centre (3.6169, 22.806) ccw
  line L3047 (1.0789, 22.869) -> (2.3365, 22.869)
  arc A3047 (2.3365, 22.869) -> (2.3365, 22.995) centre (2.3365, 22.932) ccw
  line L3048 (2.3365, 22.995) -> (1.0789, 22.995)
  arc A3048 (1.0789, 22.995) -> (1.0789, 22.869) centre (1.0789, 22.932) ccw
  line L3049 (2.4634, 22.869) -> (17.121, 22.869)
  arc A3049 (17.121, 22.869) -> (17.121, 22.995) centre (17.121, 22.932) ccw
  line L3050 (17.121, 22.995) -> (2.4634, 22.995)
  arc A3050 (2.4634, 22.995) -> (2.4634, 22.869) centre (2.4634, 22.932) ccw
  line L3051 (1.0789, 22.995) -> (1.183, 22.995)
  arc A3051 (1.183, 22.995) -> (1.183, 23.121) centre (1.183, 23.058) ccw
  line L3052 (1.183, 23.121) -> (1.0789, 23.121)
  arc A3052 (1.0789, 23.121) -> (1.0789, 22.995) centre (1.0789, 23.058) ccw
  line L3053 (2.337, 22.995) -> (2.4628, 22.995)
  arc A3053 (2.4628, 22.995) -> (2.4628, 23.121) centre (2.4628, 23.058) ccw
  line L3054 (2.4628, 23.121) -> (2.337, 23.121)
  arc A3054 (2.337, 23.121) -> (2.337, 22.995) centre (2.337, 23.058) ccw
  line L3055 (3.6169, 22.995) -> (17.121, 22.995)
  arc A3055 (17.121, 22.995) -> (17.121, 23.121) centre (17.121, 23.058) ccw
  line L3056 (17.121, 23.121) -> (3.6169, 23.121)
  arc A3056 (3.6169, 23.121) -> (3.6169, 22.995) centre (3.6169, 23.058) ccw
  line L3057 (1.0789, 23.121) -> (1.183, 23.121)
  arc A3057 (1.183, 23.121) -> (1.183, 23.247) centre (1.183, 23.184) ccw
  line L3058 (1.183, 23.247) -> (1.0789, 23.247)
  arc A3058 (1.0789, 23.247) -> (1.0789, 23.121) centre (1.0789, 23.184) ccw
  line L3059 (2.337, 23.121) -> (2.4628, 23.121)
  arc A3059 (2.4628, 23.121) -> (2.4628, 23.247) centre (2.4628, 23.184) ccw
  line L3060 (2.4628, 23.247) -> (2.337, 23.247)
  arc A3060 (2.337, 23.247) -> (2.337, 23.121) centre (2.337, 23.184) ccw
  line L3061 (3.6169, 23.121) -> (7.2806, 23.121)
  arc A3061 (7.2806, 23.121) -> (7.2806, 23.247) centre (7.2806, 23.184) ccw
  line L3062 (7.2806, 23.247) -> (3.6169, 23.247)
  arc A3062 (3.6169, 23.247) -> (3.6169, 23.121) centre (3.6169, 23.184) ccw
  line L3063 (8.1192, 23.121) -> (17.121, 23.121)
  arc A3063 (17.121, 23.121) -> (17.121, 23.247) centre (17.121, 23.184) ccw
  line L3064 (17.121, 23.247) -> (8.1192, 23.247)
  arc A3064 (8.1192, 23.247) -> (8.1192, 23.121) centre (8.1192, 23.184) ccw
  line L3065 (1.0789, 23.247) -> (1.2319, 23.247)
  arc A3065 (1.2319, 23.247) -> (1.2319, 23.373) centre (1.2319, 23.31) ccw
  line L3066 (1.2319, 23.373) -> (1.0789, 23.373)
  arc A3066 (1.0789, 23.373) -> (1.0789, 23.247) centre (1.0789, 23.31) ccw
  line L3067 (2.337, 23.247) -> (2.4628, 23.247)
  arc A3067 (2.4628, 23.247) -> (2.4628, 23.373) centre (2.4628, 23.31) ccw
  line L3068 (2.4628, 23.373) -> (2.337, 23.373)
  arc A3068 (2.337, 23.373) -> (2.337, 23.247) centre (2.337, 23.31) ccw
  line L3069 (3.5681, 23.247) -> (6.9804, 23.247)
  arc A3069 (6.9804, 23.247) -> (6.9804, 23.373) centre (6.9804, 23.31) ccw
  line L3070 (6.9804, 23.373) -> (3.5681, 23.373)
  arc A3070 (3.5681, 23.373) -> (3.5681, 23.247) centre (3.5681, 23.31) ccw
  line L3071 (8.4195, 23.247) -> (17.121, 23.247)
  arc A3071 (17.121, 23.247) -> (17.121, 23.373) centre (17.121, 23.31) ccw
  line L3072 (17.121, 23.373) -> (8.4195, 23.373)
  arc A3072 (8.4195, 23.373) -> (8.4195, 23.247) centre (8.4195, 23.31) ccw
  line L3073 (1.0789, 23.373) -> (1.2841, 23.373)
  arc A3073 (1.2841, 23.373) -> (1.2841, 23.499) centre (1.2841, 23.436) ccw
  line L3074 (1.2841, 23.499) -> (1.0789, 23.499)
  arc A3074 (1.0789, 23.499) -> (1.0789, 23.373) centre (1.0789, 23.436) ccw
  line L3075 (2.337, 23.373) -> (2.4628, 23.373)
  arc A3075 (2.4628, 23.373) -> (2.4628, 23.499) centre (2.4628, 23.436) ccw
  line L3076 (2.4628, 23.499) -> (2.337, 23.499)
  arc A3076 (2.337, 23.499) -> (2.337, 23.373) centre (2.337, 23.436) ccw
  line L3077 (3.5159, 23.373) -> (6.8544, 23.373)
  arc A3077 (6.8544, 23.373) -> (6.8544, 23.499) centre (6.8544, 23.436) ccw
  line L3078 (6.8544, 23.499) -> (3.5159, 23.499)
  arc A3078 (3.5159, 23.499) -> (3.5159, 23.373) centre (3.5159, 23.436) ccw
  line L3079 (8.5455, 23.373) -> (17.121, 23.373)
  arc A3079 (17.121, 23.373) -> (17.121, 23.499) centre (17.121, 23.436) ccw
  line L3080 (17.121, 23.499) -> (8.5455, 23.499)
  arc A3080 (8.5455, 23.499) -> (8.5455, 23.373) centre (8.5455, 23.436) ccw
  line L3081 (1.0789, 23.499) -> (1.3363, 23.499)
  arc A3081 (1.3363, 23.499) -> (1.3363, 23.625) centre (1.3363, 23.562) ccw
  line L3082 (1.3363, 23.625) -> (1.0789, 23.625)
  arc A3082 (1.0789, 23.625) -> (1.0789, 23.499) centre (1.0789, 23.562) ccw
  line L3083 (2.337, 23.499) -> (2.4628, 23.499)
  arc A3083 (2.4628, 23.499) -> (2.4628, 23.625) centre (2.4628, 23.562) ccw
  line L3084 (2.4628, 23.625) -> (2.337, 23.625)
  arc A3084 (2.337, 23.625) -> (2.337, 23.499) centre (2.337, 23.562) ccw
  line L3085 (3.4637, 23.499) -> (6.7284, 23.499)
  arc A3085 (6.7284, 23.499) -> (6.7284, 23.625) centre (6.7284, 23.562) ccw
  line L3086 (6.7284, 23.625) -> (3.4637, 23.625)
  arc A3086 (3.4637, 23.625) -> (3.4637, 23.499) centre (3.4637, 23.562) ccw
  line L3087 (8.6715, 23.499) -> (17.121, 23.499)
  arc A3087 (17.121, 23.499) -> (17.121, 23.625) centre (17.121, 23.562) ccw
  line L3088 (17.121, 23.625) -> (8.6715, 23.625)
  arc A3088 (8.6715, 23.625) -> (8.6715, 23.499) centre (8.6715, 23.562) ccw
  line L3089 (1.0789, 23.625) -> (1.417, 23.625)
  arc A3089 (1.417, 23.625) -> (1.417, 23.751) centre (1.417, 23.688) ccw
  line L3090 (1.417, 23.751) -> (1.0789, 23.751)
  arc A3090 (1.0789, 23.751) -> (1.0789, 23.625) centre (1.0789, 23.688) ccw
  line L3091 (2.337, 23.625) -> (2.4628, 23.625)
  arc A3091 (2.4628, 23.625) -> (2.4628, 23.751) centre (2.4628, 23.688) ccw
  line L3092 (2.4628, 23.751) -> (2.337, 23.751)
  arc A3092 (2.337, 23.751) -> (2.337, 23.625) centre (2.337, 23.688) ccw
  line L3093 (3.3829, 23.625) -> (6.6169, 23.625)
  arc A3093 (6.6169, 23.625) -> (6.6169, 23.751) centre (6.6169, 23.688) ccw
  line L3094 (6.6169, 23.751) -> (3.3829, 23.751)
  arc A3094 (3.3829, 23.751) -> (3.3829, 23.625) centre (3.3829, 23.688) ccw
  line L3095 (8.7829, 23.625) -> (17.121, 23.625)
  arc A3095 (17.121, 23.625) -> (17.121, 23.751) centre (17.121, 23.688) ccw
  line L3096 (17.121, 23.751) -> (8.7829, 23.751)
  arc A3096 (8.7829, 23.751) -> (8.7829, 23.625) centre (8.7829, 23.688) ccw
  line L3097 (1.0789, 23.751) -> (1.543, 23.751)
  arc A3097 (1.543, 23.751) -> (1.543, 23.877) centre (1.543, 23.814) ccw
  line L3098 (1.543, 23.877) -> (1.0789, 23.877)
  arc A3098 (1.0789, 23.877) -> (1.0789, 23.751) centre (1.0789, 23.814) ccw
  line L3099 (2.337, 23.751) -> (2.4628, 23.751)
  arc A3099 (2.4628, 23.751) -> (2.4628, 23.877) centre (2.4628, 23.814) ccw
  line L3100 (2.4628, 23.877) -> (2.337, 23.877)
  arc A3100 (2.337, 23.877) -> (2.337, 23.751) centre (2.337, 23.814) ccw
  line L3101 (3.2569, 23.751) -> (6.5647, 23.751)
  arc A3101 (6.5647, 23.751) -> (6.5647, 23.877) centre (6.5647, 23.814) ccw
  line L3102 (6.5647, 23.877) -> (3.2569, 23.877)
  arc A3102 (3.2569, 23.877) -> (3.2569, 23.751) centre (3.2569, 23.814) ccw
  line L3103 (8.8351, 23.751) -> (17.121, 23.751)
  arc A3103 (17.121, 23.751) -> (17.121, 23.877) centre (17.121, 23.814) ccw
  line L3104 (17.121, 23.877) -> (8.8351, 23.877)
  arc A3104 (8.8351, 23.877) -> (8.8351, 23.751) centre (8.8351, 23.814) ccw
  line L3105 (1.0789, 23.877) -> (1.669, 23.877)
  arc A3105 (1.669, 23.877) -> (1.669, 24.003) centre (1.669, 23.94) ccw
  line L3106 (1.669, 24.003) -> (1.0789, 24.003)
  arc A3106 (1.0789, 24.003) -> (1.0789, 23.877) centre (1.0789, 23.94) ccw
  line L3107 (2.337, 23.877) -> (2.4628, 23.877)
  arc A3107 (2.4628, 23.877) -> (2.4628, 24.003) centre (2.4628, 23.94) ccw
  line L3108 (2.4628, 24.003) -> (2.337, 24.003)
  arc A3108 (2.337, 24.003) -> (2.337, 23.877) centre (2.337, 23.94) ccw
  line L3109 (3.1309, 23.877) -> (6.5125, 23.877)
  arc A3109 (6.5125, 23.877) -> (6.5125, 24.003) centre (6.5125, 23.94) ccw
  line L3110 (6.5125, 24.003) -> (3.1309, 24.003)
  arc A3110 (3.1309, 24.003) -> (3.1309, 23.877) centre (3.1309, 23.94) ccw
  line L3111 (8.8873, 23.877) -> (17.121, 23.877)
  arc A3111 (17.121, 23.877) -> (17.121, 24.003) centre (17.121, 23.94) ccw
  line L3112 (17.121, 24.003) -> (8.8873, 24.003)
  arc A3112 (8.8873, 24.003) -> (8.8873, 23.877) centre (8.8873, 23.94) ccw
  line L3113 (1.0789, 24.003) -> (1.9143, 24.003)
  arc A3113 (1.9143, 24.003) -> (1.9143, 24.129) centre (1.9143, 24.066) ccw
  line L3114 (1.9143, 24.129) -> (1.0789, 24.129)
  arc A3114 (1.0789, 24.129) -> (1.0789, 24.003) centre (1.0789, 24.066) ccw
  line L3115 (2.337, 24.003) -> (2.4628, 24.003)
  arc A3115 (2.4628, 24.003) -> (2.4628, 24.129) centre (2.4628, 24.066) ccw
  line L3116 (2.4628, 24.129) -> (2.337, 24.129)
  arc A3116 (2.337, 24.129) -> (2.337, 24.003) centre (2.337, 24.066) ccw
  line L3117 (2.8857, 24.003) -> (6.4603, 24.003)
  arc A3117 (6.4603, 24.003) -> (6.4603, 24.129) centre (6.4603, 24.066) ccw
  line L3118 (6.4603, 24.129) -> (2.8857, 24.129)
  arc A3118 (2.8857, 24.129) -> (2.8857, 24.003) centre (2.8857, 24.066) ccw
  line L3119 (8.9395, 24.003) -> (17.121, 24.003)
  arc A3119 (17.121, 24.003) -> (17.121, 24.129) centre (17.121, 24.066) ccw
  line L3120 (17.121, 24.129) -> (8.9395, 24.129)
  arc A3120 (8.9395, 24.129) -> (8.9395, 24.003) centre (8.9395, 24.066) ccw
  line L3121 (1.0789, 24.129) -> (6.4346, 24.129)
  arc A3121 (6.4346, 24.129) -> (6.4346, 24.255) centre (6.4346, 24.192) ccw
  line L3122 (6.4346, 24.255) -> (1.0789, 24.255)
  arc A3122 (1.0789, 24.255) -> (1.0789, 24.129) centre (1.0789, 24.192) ccw
  line L3123 (8.9653, 24.129) -> (17.121, 24.129)
  arc A3123 (17.121, 24.129) -> (17.121, 24.255) centre (17.121, 24.192) ccw
  line L3124 (17.121, 24.255) -> (8.9653, 24.255)
  arc A3124 (8.9653, 24.255) -> (8.9653, 24.129) centre (8.9653, 24.192) ccw
  line L3125 (1.0789, 24.255) -> (6.4346, 24.255)
  arc A3125 (6.4346, 24.255) -> (6.4346, 24.381) centre (6.4346, 24.318) ccw
  line L3126 (6.4346, 24.381) -> (1.0789, 24.381)
  arc A3126 (1.0789, 24.381) -> (1.0789, 24.255) centre (1.0789, 24.318) ccw
  line L3127 (8.9653, 24.255) -> (17.121, 24.255)
  arc A3127 (17.121, 24.255) -> (17.121, 24.381) centre (17.121, 24.318) ccw
  line L3128 (17.121, 24.381) -> (8.9653, 24.381)
  arc A3128 (8.9653, 24.381) -> (8.9653, 24.255) centre (8.9653, 24.318) ccw
  line L3129 (1.0789, 24.381) -> (6.4346, 24.381)
  arc A3129 (6.4346, 24.381) -> (6.4346, 24.507) centre (6.4346, 24.444) ccw
  line L3130 (6.4346, 24.507) -> (1.0789, 24.507)
  arc A3130 (1.0789, 24.507) -> (1.0789, 24.381) centre (1.0789, 24.444) ccw
  line L3131 (8.9653, 24.381) -> (17.121, 24.381)
  arc A3131 (17.121, 24.381) -> (17.121, 24.507) centre (17.121, 24.444) ccw
  line L3132 (17.121, 24.507) -> (8.9653, 24.507)
  arc A3132 (8.9653, 24.507) -> (8.9653, 24.381) centre (8.9653, 24.444) ccw
  line L3133 (1.0789, 24.507) -> (6.4346, 24.507)
  arc A3133 (6.4346, 24.507) -> (6.4346, 24.633) centre (6.4346, 24.57) ccw
  line L3134 (6.4346, 24.633) -> (1.0789, 24.633)
  arc A3134 (1.0789, 24.633) -> (1.0789, 24.507) centre (1.0789, 24.57) ccw
  line L3135 (8.9653, 24.507) -> (17.121, 24.507)
  arc A3135 (17.121, 24.507) -> (17.121, 24.633) centre (17.121, 24.57) ccw
  line L3136 (17.121, 24.633) -> (8.9653, 24.633)
  arc A3136 (8.9653, 24.633) -> (8.9653, 24.507) centre (8.9653, 24.57) ccw
  line L3137 (1.0789, 24.633) -> (6.4613, 24.633)
  arc A3137 (6.4613, 24.633) -> (6.4613, 24.759) centre (6.4613, 24.696) ccw
  line L3138 (6.4613, 24.759) -> (1.0789, 24.759)
  arc A3138 (1.0789, 24.759) -> (1.0789, 24.633) centre (1.0789, 24.696) ccw
  line L3139 (8.9387, 24.633) -> (17.121, 24.633)
  arc A3139 (17.121, 24.633) -> (17.121, 24.759) centre (17.121, 24.696) ccw
  line L3140 (17.121, 24.759) -> (8.9387, 24.759)
  arc A3140 (8.9387, 24.759) -> (8.9387, 24.633) centre (8.9387, 24.696) ccw
  line L3141 (1.0789, 24.759) -> (6.5135, 24.759)
  arc A3141 (6.5135, 24.759) -> (6.5135, 24.885) centre (6.5135, 24.822) ccw
  line L3142 (6.5135, 24.885) -> (1.0789, 24.885)
  arc A3142 (1.0789, 24.885) -> (1.0789, 24.759) centre (1.0789, 24.822) ccw
  line L3143 (8.8865, 24.759) -> (17.121, 24.759)
  arc A3143 (17.121, 24.759) -> (17.121, 24.885) centre (17.121, 24.822) ccw
  line L3144 (17.121, 24.885) -> (8.8865, 24.885)
  arc A3144 (8.8865, 24.885) -> (8.8865, 24.759) centre (8.8865, 24.822) ccw
  line L3145 (1.0789, 24.885) -> (6.5657, 24.885)
  arc A3145 (6.5657, 24.885) -> (6.5657, 25.011) centre (6.5657, 24.948) ccw
  line L3146 (6.5657, 25.011) -> (1.0789, 25.011)
  arc A3146 (1.0789, 25.011) -> (1.0789, 24.885) centre (1.0789, 24.948) ccw
  line L3147 (8.8343, 24.885) -> (17.121, 24.885)
  arc A3147 (17.121, 24.885) -> (17.121, 25.011) centre (17.121, 24.948) ccw
  line L3148 (17.121, 25.011) -> (8.8343, 25.011)
  arc A3148 (8.8343, 25.011) -> (8.8343, 24.885) centre (8.8343, 24.948) ccw
  line L3149 (1.0789, 25.011) -> (6.6178, 25.011)
  arc A3149 (6.6178, 25.011) -> (6.6178, 25.137) centre (6.6178, 25.074) ccw
  line L3150 (6.6178, 25.137) -> (1.0789, 25.137)
  arc A3150 (1.0789, 25.137) -> (1.0789, 25.011) centre (1.0789, 25.074) ccw
  line L3151 (8.7822, 25.011) -> (17.121, 25.011)
  arc A3151 (17.121, 25.011) -> (17.121, 25.137) centre (17.121, 25.074) ccw
  line L3152 (17.121, 25.137) -> (8.7822, 25.137)
  arc A3152 (8.7822, 25.137) -> (8.7822, 25.011) centre (8.7822, 25.074) ccw
  line L3153 (1.0789, 25.137) -> (6.7305, 25.137)
  arc A3153 (6.7305, 25.137) -> (6.7305, 25.263) centre (6.7305, 25.2) ccw
  line L3154 (6.7305, 25.263) -> (1.0789, 25.263)
  arc A3154 (1.0789, 25.263) -> (1.0789, 25.137) centre (1.0789, 25.2) ccw